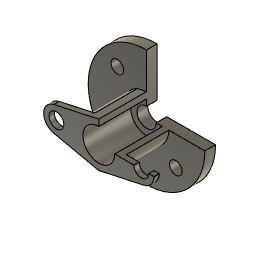
Sketch23_Final v0 (Autodesk Fusion 360 design; units mm, degrees)
Autodesk Fusion 360 part; units mm, degrees
note: some values were not read from the file. Chosen so that the rebuilt part matches the saved one: which face or edge a step refers to. Set by a fixed rule: which sketch regions a step uses.
sketch "Sketch1" plane through (0, 0, 0) normal (0, 1, 0) x (1, 0, 0)
  circle A0 centre (0, 0) radius 55
  circle A1 centre (0, 0) radius 15
  line L0 (0, 0) -> (38.8909, 38.8909)
  line L1 (0, 0) -> (55, 0) construction
  line L2 (0, -70) -> (0, 0)
  line L3 (0, 0) -> (70, 0)
  line L4 (70, 0) -> (70, -70)
  line L5 (70, -70) -> (0, -70)
  circle A2 centre (0, 0) radius 9
  dimension "d1" = 110
  dimension "d2" = 30
  dimension "d3" = 45
  dimension "d24" = 18
  constraint coincident A0.centre A1.centre
  constraint concentric A0 A1
  constraint horizontal L1
  constraint perpendicular L1 L2
  constraint perpendicular L2 L3
  constraint perpendicular L1 L4
  constraint perpendicular L2 L5
  constraint concentric A0 A2
  measures "d1" diameter of A0
  measures "d2" diameter of A1
  measures "d3" angle of L0 L1
  measures "d24" diameter of A2
ref_plane "WorkPlane1" through (0, -45, 0) normal (0, 1, 0) x (1, 0, 0)
sketch "Sketch2" plane through (0, -45, 0) normal (0, 1, 0) x (1, 0, 0)
  circle A0 centre (0, 0) radius 15
  circle A1 centre (-40, 0) radius 7
  line L0 (0, 0) -> (0, -21)
  line L1 (0, 0) -> (0, 21)
  line L2 (0, -21) -> (-42.5555, -11.7247)
  line L3 (0, 21) -> (-42.5555, 11.7247)
  arc A2 (-40, 12) -> (-40, -12) centre (-40, 0) ccw
  arc A3 (-8.739, -19.0953) -> (-8.739, 19.0953) centre (0, 0) ccw
  line L4 (0, 21) -> (42.5555, 11.7247)
  arc A4 (40, -12) -> (40, 12) centre (40, 0) ccw
  circle A5 centre (40, 0) radius 7
  line L5 (0, -21) -> (42.5555, -11.7247)
  arc A6 (8.739, 19.0953) -> (8.739, -19.0953) centre (0, 0) ccw
  dimension "d5" = 30
  dimension "d6" = 42
  dimension "d7" = 40
  dimension "d8" = 14
  dimension "d9" = 24
  dimension "d10" = 12
  constraint coincident A0.centre L0.start
  constraint concentric A1 A2
  constraint coincident L0.end A3
  constraint coincident L1.end A3
  constraint coincident L2.end A2
  constraint tangent L2 A2
  constraint coincident L3.end A2
  constraint tangent L3 A2
  constraint coincident L2 A3.start
  constraint coincident L3 A3.end
  constraint symmetric A1 L0 A5
  constraint symmetric A2.end L0 A4.start
  constraint symmetric A2.start L0 A4.end
  constraint symmetric L2.start L0 L5.start
  constraint symmetric L0 L1.end L3.start
  constraint symmetric L0 L2.end L5.end
  constraint symmetric L0 L3.end L4.end
  constraint symmetric L0 A2 A4
  constraint symmetric L0 A3.start A6.end
  constraint symmetric L0 A3 A6
  constraint symmetric L0 A3.end A6.start
  measures "d5" diameter of A0
  measures "d6" diameter of A3
  measures "d7" distance of A0.centre A1.centre
  measures "d8" diameter of A1
  measures "d9" diameter of A2
  measures "d10" distance of A1.centre A2.start
extrude "Extrude1" add sketch "Sketch1" along normal blind 10 contours A0 A1 L0 L3 | A0 A1 L2 L3 | A0 A1 L0 L2
extrude "Extrude2" add sketch "Sketch2" along normal blind 45 contours A0 L0 L1 A3 L4 L5 | A0 L0 L1 L2 L3 A6
extrude "Extrude3" add sketch "Sketch2" along normal blind 5 contours L2 L3 A2 A6 | A3 L4 A4 L5
hole "Hole1" at (27.5605, 0, -27.5276) direction (0, 1, 0) diameter 12 depth 10 tip angle 118
pattern_circular "C-Pattern1" count 4 over 360 about axis through (0, 1.75, 0) along (0, 1, 0) of "Hole1"
extrude "Extrude4" cut sketch "Sketch1" along normal mid plane 90 contours A0 L2 L3 L4 L5 | A0 A1 L2 L3 | A1 L2 L3 A2 | L2 L3 A2
extrude "Extrude5" add sketch "Sketch1" along normal blind 10 contours A1 L0 L3 A2 | A1 L2 L3 A2 | A1 L0 L2 A2
extrude "Extrude6" cut sketch "Sketch1" along normal blind 10 contours A1 L2 L3 A2
